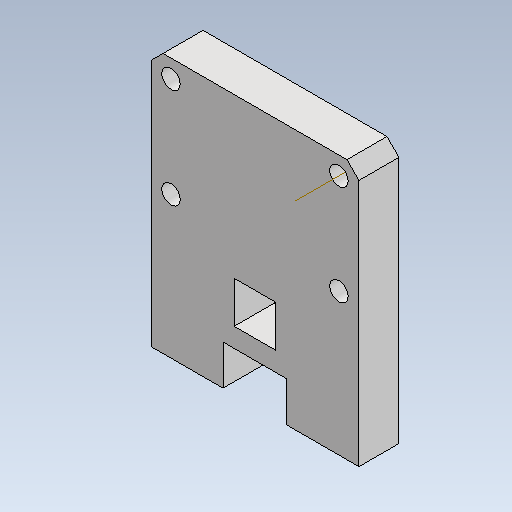
# Autodesk Inventor part: camera-bracket
Saved by Autodesk Inventor 2025 (Build 290162000, 162)
## iProperties
Created: 2025-08-26
Part Number: camera-bracket
Material: Generic
Document SubType Name: Modeling
Designer: HP
Density: 1 g/cm^3
Appearance: Default
Author: HP
Autodesk Inventor part; units mm, degrees
ref_plane "YZ Plane" through (0, 0, 0) normal (1, 0, 0) x (0, 1, 0)
ref_plane "XZ Plane" through (0, 0, 0) normal (0, 1, 0) x (-1, 0, 0)
ref_plane "XY Plane" through (0, 0, 0) normal (0, 0, 1) x (1, 0, 0)
sketch "Sketch1" plane through (0, 0, 0) normal (0, 0, 1) x (1, 0, 0)
  line L0 (-13, -16.25) -> (13, -16.25)
  line L1 (13, -16.25) -> (13, 16.25)
  line L2 (13, 16.25) -> (-13, 16.25)
  line L3 (-13, 16.25) -> (-13, -16.25)
  line L4 (-13, -16.25) -> (13, 16.25) construction
  line L5 (13, -16.25) -> (-13, 16.25) construction
  line L6 (-10.5, 1.5) -> (10.5, 1.5) construction
  line L7 (10.5, 1.5) -> (10.5, 14) construction
  line L8 (10.5, 14) -> (-10.5, 14) construction
  line L9 (-10.5, 14) -> (-10.5, 1.5) construction
  line L10 (-10.5, 1.5) -> (10.5, 14) construction
  line L11 (10.5, 1.5) -> (-10.5, 14) construction
  circle A0 centre (-10.5, 14) radius 1.15
  circle A1 centre (10.5, 14) radius 1.15
  circle A2 centre (10.5, 1.5) radius 1.15
  circle A3 centre (-10.5, 1.5) radius 1.15
  line L12 (-13, -11.25) -> (-4, -11.25) construction
  line L13 (-4, -11.25) -> (-4, -16.25)
  line L14 (-4, -16.25) -> (-13, -16.25)
  line L15 (-13, -16.25) -> (-13, -11.25)
  line L16 (-13, -11.25) -> (-4, -16.25) construction
  line L17 (-4, -11.25) -> (-13, -16.25) construction
  line L18 (4, -11.25) -> (13, -11.25) construction
  line L19 (13, -11.25) -> (13, -16.25)
  line L20 (13, -16.25) -> (4, -16.25)
  line L21 (4, -16.25) -> (4, -11.25)
  line L22 (4, -11.25) -> (13, -16.25) construction
  line L23 (13, -11.25) -> (4, -16.25) construction
  line L24 (-4, -11.25) -> (4, -11.25)
  line L25 (-2.6, -8.85) -> (2.6, -8.85)
  line L26 (2.6, -8.85) -> (2.6, -3.65)
  line L27 (2.6, -3.65) -> (-2.6, -3.65)
  line L28 (-2.6, -3.65) -> (-2.6, -8.85)
  line L29 (-2.6, -8.85) -> (2.6, -3.65) construction
  line L30 (2.6, -8.85) -> (-2.6, -3.65) construction
  point P0 (0, 0)
  point P1 (0, 7.75)
  point P2 (0, 7.75)
  point P3 (-8.5, -13.75)
  point P4 (8.5, -13.75)
  point P5 (0, -11.25)
  point P6 (0, -16.25)
  point P7 (4, -16.25)
  point P8 (0, -6.25)
  dimension "d0" = 12.5
  dimension "d1" = 21
  dimension "d2" = 2.3
  dimension "d3" = 2.3
  dimension "d4" = 2.3
  dimension "d5" = 2.3
  dimension "d6" = 26
  dimension "d7" = 32.5
  dimension "d9" = 5
  dimension "d10" = 9
  dimension "d11" = 5
  dimension "d12" = 9
  dimension "d17" = 5.2
  dimension "d18" = 5.2
  dimension "d19" = 10
  dimension "d20" = 8.5
  constraints: 62 end point, 12 midpoint, 10 parallel, 5 horizontal, 5 perpendicular, 4 centre point, 4 coincident, 3 vertical alignment, 2 collinear, 1 horizontal alignment
  measures "d0" distance between parallel lines of L6 L8
  measures "d1" distance between parallel lines of L7 L9
  measures "d2" diameter of A1
  measures "d3" diameter of A0
  measures "d4" diameter of A2
  measures "d5" diameter of A3
  measures "d6" distance between parallel lines of L1 L3
  measures "d7" distance between parallel lines of L0 L2
  measures "d9" distance between parallel lines of L14 L12
  measures "d10" distance between parallel lines of L15 L13
  measures "d11" distance between parallel lines of L20 L18
  measures "d12" distance between parallel lines of L21 L19
  measures "d17" distance between parallel lines of L25 L27
  measures "d18" distance between parallel lines of L26 L28
  measures "d19" distance from line of L0 point (0, -6.25)
  measures "d20" distance from line of point (0, 7.75) L2
extrude "Extrusion1" add sketch "Sketch1" along normal blind 5 contours L3 L2 L1 L0 L21 L24 L13
chamfer "Chamfer1" distance 1.5 angle 45 2 edges at (13, 16.25, 2.5) (-13, 16.25, 2.5)
equation "\"d2\" = d3"
equation "\"d4\" = d2"
equation "\"d5\" = d4"
equation "\"d11\" = d9"
equation "\"d12\" = d10"
body "Solid1"
